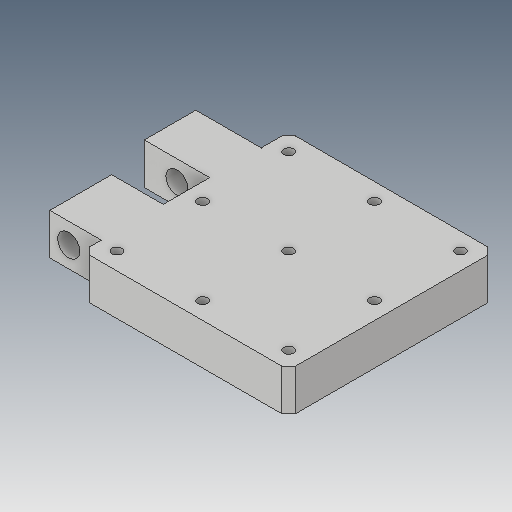
# Autodesk Inventor part: 00_XY_stage-CHUO_SEIKI_LD-647-R1-Top
Saved by Autodesk Inventor 2019 (Build 230136000, 136)
## iProperties
Created: 2019-05-02
Part Number: 00_XY_stage-CHUO_SEIKI_LD-647-R1-Top
Material: Generic
Document SubType Name: Modeling
Designer: diederichbenedict
Density: 1 g/cm^3
Appearance: Default
Author: diederichbenedict
Autodesk Inventor part; units mm, degrees
ref_plane "YZ Plane" through (0, 0, 0) normal (1, 0, 0) x (0, 1, 0)
ref_plane "XZ Plane" through (0, 0, 0) normal (0, 1, 0) x (-1, 0, 0)
sketch "Sketch1" plane through (0, 0, 0) normal (0, 1, 0) x (-1, 0, 0)
  line L0 (-30, -30) -> (30, -30)
  line L1 (30, -30) -> (30, 30)
  line L2 (30, 30) -> (-30, 30)
  line L3 (-30, 30) -> (-30, -30)
  line L4 (-30, -30) -> (30, 30) construction
  line L5 (30, -30) -> (-30, 30) construction
  circle A0 centre (0, 0) radius 7.5
  dimension "d0" = 60
  dimension "d1" = 60
  dimension "d13" = 15
  constraints: 12 end point, 2 midpoint, 2 parallel, 1 centre point, 1 coincident, 1 horizontal, 1 perpendicular
  measures "d0" distance of L2.end L1.end
  measures "d1" distance of L1.end L0.end
  measures "d13" diameter of A0
extrude "Extrusion1" add sketch "Sketch1" along normal blind 12 contours L3 L2 L1 L0 | A0
sketch "Sketch2" plane through (0, 12, 0) normal (0, 1, 0) x (1, 0, 0)
  line L0 (30, 30) -> (-30, 30) projected
  line L1 (-30, 30) -> (-30, -30) projected
  line L2 (-30, -30) -> (30, -30) projected
  line L3 (30, -30) -> (30, 30) projected
  line L4 (25, -25) -> (-25, -25)
  line L5 (-25, -25) -> (-25, 25)
  line L6 (-25, 25) -> (25, 25)
  line L7 (25, 25) -> (25, -25)
  line L8 (25, -25) -> (-25, 25) construction
  line L9 (-25, -25) -> (25, 25) construction
  line L10 (0, -25) -> (0, 25)
  line L11 (-25, 0) -> (25, 0)
  point P0 (0, 0)
  point P1 (0, 0)
  dimension "d4" = 50
  dimension "d5" = 50
  constraints: 16 end point, 6 midpoint, 5 coincident, 2 parallel, 1 horizontal, 1 perpendicular
  measures "d4" distance of L5.end L6.end
  measures "d5" distance of L4.end L5.end
hole "Hole1" at (-25, 12, 25) at (-25, 12, -25) at (25, 12, -25) at (25, 12, 25) at (0, 12, 25) at (0, 12, 0) at (-25, 12, 0) at (0, 12, -25) at (25, 12, 0) direction (0, -1, 0) diameter 2.9 depth 10 tip angle 118
chamfer "Chamfer1" distance 2 angle 45 4 edges at (30, 6, 30) (30, 6, -30) (-30, 6, -30) (-30, 6, 30)
sketch "Sketch3" plane through (0, 12, 0) normal (0, 1, 0) x (1, 0, 0)
  line L0 (-28, -30) -> (-30, -28) projected
  line L1 (-28, -30) -> (28, -30) projected
  line L2 (30, -28) -> (28, -30) projected
  line L3 (30, -28) -> (30, 28) projected
  line L4 (28, 30) -> (30, 28) projected
  line L5 (28, 30) -> (-28, 30) projected
  line L6 (-30, 28) -> (-28, 30) projected
  line L7 (-30, 28) -> (-30, -28) projected
  circle A0 centre (0, 25) radius 1.45 projected
  circle A1 centre (0, 0) radius 1.45 projected
  circle A2 centre (25, -25) radius 1.45 projected
  circle A3 centre (-25, 25) radius 1.45 projected
  circle A4 centre (-25, -25) radius 1.45 projected
  circle A5 centre (25, 25) radius 1.45 projected
  circle A6 centre (0, -25) radius 1.45 projected
  circle A7 centre (-25, 0) radius 1.45 projected
  circle A8 centre (25, 0) radius 1.45 projected
  line L8 (-30, 28) -> (-30, -28) projected
  line L9 (-30, -24.5) -> (-45, -24.5)
  line L10 (-45, -24.5) -> (-45, -6.5)
  line L11 (-45, -6.5) -> (-30, -6.5)
  line L12 (-30, -6.5) -> (-30, -24.5)
  line L13 (-30, 7) -> (-45, 7)
  line L14 (-45, 7) -> (-45, 22)
  line L15 (-45, 22) -> (-30, 22)
  line L16 (-30, 22) -> (-30, 7)
  line L17 (-45, 7) -> (-49, 7)
  line L18 (-49, 7) -> (-49, 22)
  line L19 (-49, 22) -> (-45, 22)
  line L20 (-45, 22) -> (-45, 7)
  dimension "d17" = 15
  dimension "d18" = 18
  dimension "d19" = 5.5
  dimension "d20" = 15
  dimension "d21" = 8
  dimension "d22" = 19
  constraints: 24 end point, 6 parallel, 3 horizontal, 3 perpendicular, 3 point on line
  measures "d17" distance between parallel lines of L10 L7
  measures "d18" distance between parallel lines of L11 L9
  measures "d19" distance between parallel lines of L9 L1
  measures "d20" distance between parallel lines of L15 L13
  measures "d21" distance between parallel lines of L5 L15
  measures "d22" distance between parallel lines of L7 L18
ref_plane "Work Plane1" through (-30, 0, -30) normal (0, 1, 0) x (0, 0, 1)
extrude "Extrusion2" add sketch "Sketch3" against normal up to surface (12 mm away) contours L9 L10 L11 L7 | L13 L14 L15 L7 | L17 L18 L19 L14
sketch "Sketch4" plane through (-30, 12, -22) normal (0, 0, -1) x (-1, 0, 0)
  line L0 (15, 0) -> (15, -12) projected
  line L1 (19, -12) -> (0, -12) projected
  line L2 (19, 0) -> (19, -12) projected
  line L3 (0, 0) -> (19, 0) projected
  line L4 (0, -12) -> (0, 0) projected
  circle A0 centre (9.5, -6) radius 3.2291
  point P0 (-30, -12)
  constraints: 1 centre point
extrude "Extrusion3" cut sketch "Sketch4" against normal through all contours A0
body "Solid1"
